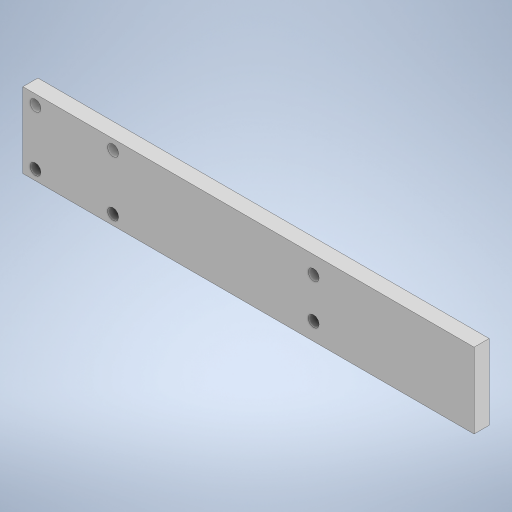
# Autodesk Inventor part: slider_to_cutter_part
Saved by Autodesk Inventor 2024.3 (Build 283343000, 343)
## iProperties
Created: 2025-06-10
Part Number: slider_to_cutter_part
Material: 一般
Document SubType Name: Modeling
Designer: hikou
Density: 1 g/cm^3
Appearance: 既定
Author: hikou
Autodesk Inventor part; units mm, degrees
ref_plane "YZ Plane" through (0, 0, 0) normal (1, 0, 0) x (0, 1, 0)
ref_plane "XZ Plane" through (0, 0, 0) normal (0, 1, 0) x (-1, 0, 0)
ref_plane "XY Plane" through (0, 0, 0) normal (0, 0, 1) x (1, 0, 0)
sketch "スケッチ1" plane through (0, 0, 0) normal (0, 0, 1) x (1, 0, 0)
  line L0 (-45, -7.5) -> (45, -7.5)
  line L1 (45, -7.5) -> (45, 7.5)
  line L2 (45, 7.5) -> (-45, 7.5)
  line L3 (-45, 7.5) -> (-45, -7.5)
  line L4 (-45, -7.5) -> (45, 7.5) construction
  line L5 (45, -7.5) -> (-45, 7.5) construction
  point P0 (0, 0)
  dimension "d0" = 90
  dimension "d1" = 15
  constraints: 12 end point, 2 midpoint, 2 parallel, 1 horizontal, 1 perpendicular
  measures "d0" distance of L1.end L2.end
  measures "d1" distance of L0.end L1.end
extrude "押し出し1" add sketch "スケッチ1" along normal mid plane 3
sketch "スケッチ2" plane through (0, 0, 1.5) normal (0, 0, 1) x (1, 0, 0)
  line L0 (-45, 7.5) -> (-45, -7.5) projected
  line L1 (0, 0) -> (-7.3146, 0)
  point P0 (-42.5, 5.5)
  point P1 (-27, 5.5)
  point P2 (-42.5, -5.5)
  point P3 (-27, -5.5)
  dimension "d4" = 2.5
  dimension "d5" = 15.5
  dimension "d6" = 5.5
  dimension "d7" = 5.5
  constraints: 2 end point, 2 symmetric about line, 1 horizontal
  measures "d4" distance from line of L0 point (-42.5, 5.5)
  measures "d5" distance of point (-27, 5.5) point (-42.5, 5.5)
  measures "d6" vertical distance of L1.start point (-42.5, 5.5)
  measures "d7" vertical distance of L1.start point (-27, 5.5)
hole "穴1" at (-42.5, 5.5, 1.5) at (-27, 5.5, 1.5) at (-42.5, -5.5, 1.5) at (-27, -5.5, 1.5) direction (0, 0, -1) diameter 2.2 end through all
sketch "スケッチ3" plane through (0, 0, 1.5) normal (0, 0, 1) x (1, 0, 0)
  circle A0 centre (-27, 5.5) radius 1.1 projected
  circle A1 centre (-27, -5.5) radius 1.1 projected
  point P0 (0, 0)
  point P1 (13, 4)
  point P2 (13, -4)
  dimension "d15" = 40
  dimension "d16" = 4
  dimension "d17" = 4
  dimension "d18" = 40
  measures "d15" horizontal distance of A0.centre point (13, 4)
  measures "d16" vertical distance of point (0, 0) point (13, 4)
  measures "d17" vertical distance of point (0, 0) point (13, -4)
  measures "d18" horizontal distance of A1.centre point (13, -4)
hole "穴2" at (13, 4, 1.5) at (13, -4, 1.5) direction (0, 0, -1) diameter 2.2 end through all
equation "\"d7\" = d6"
equation "\"d17\" = d16"
